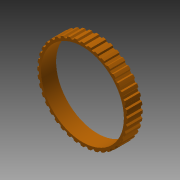
# Autodesk Inventor part: 6plactiontread
Saved by Autodesk Inventor 2013 (Build 170138000, 138)
## iProperties
Created: 2013-01-18
Part Number: 6plactiontread
Material: Rubber
Document SubType Name: Modeling
Designer: Moses
Density: 0.93 g/cm^3
Mass: 50.6346 g
Surface Area: 286.772 cm^2
Volume: 54.4458 cm^3
Author: Moses
Autodesk Inventor part; units mm, degrees
ref_plane "YZ Plane" through (0, 0, 0) normal (1, 0, 0) x (0, 1, 0)
ref_plane "XZ Plane" through (0, 0, 0) normal (0, 1, 0) x (-1, 0, 0)
ref_plane "XY Plane" through (0, 0, 0) normal (0, 0, 1) x (1, 0, 0)
sketch "Sketch1" plane through (0, 0, 0) normal (0, 0, 1) x (1, 0, 0)
  arc A0 (2.4972, 77.4343) -> (-2.4972, 77.4343) centre (0, 0) ccw
  line L0 (-3.9666, 74.7221) -> (-2.4972, 77.4343)
  line L1 (-7.7713, 74.4227) -> (-3.9666, 74.7221)
  line L2 (-9.647, 76.8716) -> (-7.7713, 74.4227)
  arc A1 (-9.647, 76.8716) -> (-14.5798, 76.0903) centre (0, 0) ccw
  line L3 (-15.6069, 73.1817) -> (-14.5798, 76.0903)
  line L4 (-19.3179, 72.2907) -> (-15.6069, 73.1817)
  line L5 (-21.5536, 74.4161) -> (-19.3179, 72.2907)
  arc A2 (-21.5536, 74.4161) -> (-26.3034, 72.8727) centre (0, 0) ccw
  line L6 (-26.8629, 69.8392) -> (-26.3034, 72.8727)
  line L7 (-30.3889, 68.3787) -> (-26.8629, 69.8392)
  line L8 (-32.9295, 70.1282) -> (-30.3889, 68.3787)
  arc A3 (-32.9295, 70.1282) -> (-37.3794, 67.8608) centre (0, 0) ccw
  line L9 (-37.4574, 64.7771) -> (-37.3794, 67.8608)
  line L10 (-40.7115, 62.783) -> (-37.4574, 64.7771)
  line L11 (-43.4945, 64.1135) -> (-40.7115, 62.783)
  arc A4 (-43.4945, 64.1135) -> (-47.535, 61.1779) centre (0, 0) ccw
  line L12 (-47.1296, 58.12) -> (-47.535, 61.1779)
  line L13 (-50.0317, 55.6414) -> (-47.1296, 58.12)
  line L14 (-52.9886, 56.5201) -> (-50.0317, 55.6414)
  arc A5 (-52.9886, 56.5201) -> (-56.5201, 52.9886) centre (0, 0) ccw
  line L15 (-55.6414, 50.0317) -> (-56.5201, 52.9886)
  line L16 (-58.12, 47.1296) -> (-55.6414, 50.0317)
  line L17 (-61.1779, 47.535) -> (-58.12, 47.1296)
  arc A6 (-61.1779, 47.535) -> (-64.1135, 43.4945) centre (0, 0) ccw
  line L18 (-62.783, 40.7115) -> (-64.1135, 43.4945)
  line L19 (-64.7771, 37.4574) -> (-62.783, 40.7115)
  line L20 (-67.8608, 37.3794) -> (-64.7771, 37.4574)
  arc A7 (-67.8608, 37.3794) -> (-70.1282, 32.9295) centre (0, 0) ccw
  line L21 (-68.3787, 30.3889) -> (-70.1282, 32.9295)
  line L22 (-69.8392, 26.8629) -> (-68.3787, 30.3889)
  line L23 (-72.8727, 26.3034) -> (-69.8392, 26.8629)
  arc A8 (-72.8727, 26.3034) -> (-74.4161, 21.5536) centre (0, 0) ccw
  line L24 (-72.2907, 19.3179) -> (-74.4161, 21.5536)
  line L25 (-73.1817, 15.6069) -> (-72.2907, 19.3179)
  line L26 (-76.0903, 14.5798) -> (-73.1817, 15.6069)
  arc A9 (-76.0903, 14.5798) -> (-76.8716, 9.647) centre (0, 0) ccw
  line L27 (-74.4227, 7.7713) -> (-76.8716, 9.647)
  line L28 (-74.7221, 3.9666) -> (-74.4227, 7.7713)
  line L29 (-77.4343, 2.4972) -> (-74.7221, 3.9666)
  arc A10 (-77.4343, 2.4972) -> (-77.4343, -2.4972) centre (0, 0) ccw
  line L30 (-74.7221, -3.9666) -> (-77.4343, -2.4972)
  line L31 (-74.4227, -7.7713) -> (-74.7221, -3.9666)
  line L32 (-76.8716, -9.647) -> (-74.4227, -7.7713)
  arc A11 (-76.8716, -9.647) -> (-76.0903, -14.5798) centre (0, 0) ccw
  line L33 (-73.1817, -15.6069) -> (-76.0903, -14.5798)
  line L34 (-72.2907, -19.3179) -> (-73.1817, -15.6069)
  line L35 (-74.4161, -21.5536) -> (-72.2907, -19.3179)
  arc A12 (-74.4161, -21.5536) -> (-72.8727, -26.3034) centre (0, 0) ccw
  line L36 (-69.8392, -26.8629) -> (-72.8727, -26.3034)
  line L37 (-68.3787, -30.3889) -> (-69.8392, -26.8629)
  line L38 (-70.1282, -32.9295) -> (-68.3787, -30.3889)
  arc A13 (-70.1282, -32.9295) -> (-67.8608, -37.3794) centre (0, 0) ccw
  line L39 (-64.7771, -37.4574) -> (-67.8608, -37.3794)
  line L40 (-62.783, -40.7115) -> (-64.7771, -37.4574)
  line L41 (-64.1135, -43.4945) -> (-62.783, -40.7115)
  arc A14 (-64.1135, -43.4945) -> (-61.1779, -47.535) centre (0, 0) ccw
  line L42 (-58.12, -47.1296) -> (-61.1779, -47.535)
  line L43 (-55.6414, -50.0317) -> (-58.12, -47.1296)
  line L44 (-56.5201, -52.9886) -> (-55.6414, -50.0317)
  arc A15 (-56.5201, -52.9886) -> (-52.9886, -56.5201) centre (0, 0) ccw
  line L45 (-50.0317, -55.6414) -> (-52.9886, -56.5201)
  line L46 (-47.1296, -58.12) -> (-50.0317, -55.6414)
  line L47 (-47.535, -61.1779) -> (-47.1296, -58.12)
  arc A16 (-47.535, -61.1779) -> (-43.4945, -64.1135) centre (0, 0) ccw
  line L48 (-40.7115, -62.783) -> (-43.4945, -64.1135)
  line L49 (-37.4574, -64.7771) -> (-40.7115, -62.783)
  line L50 (-37.3794, -67.8608) -> (-37.4574, -64.7771)
  arc A17 (-37.3794, -67.8608) -> (-32.9295, -70.1282) centre (0, 0) ccw
  line L51 (-30.3889, -68.3787) -> (-32.9295, -70.1282)
  line L52 (-26.8629, -69.8392) -> (-30.3889, -68.3787)
  line L53 (-26.3034, -72.8727) -> (-26.8629, -69.8392)
  arc A18 (-26.3034, -72.8727) -> (-21.5536, -74.4161) centre (0, 0) ccw
  line L54 (-19.3179, -72.2907) -> (-21.5536, -74.4161)
  line L55 (-15.6069, -73.1817) -> (-19.3179, -72.2907)
  line L56 (-14.5798, -76.0903) -> (-15.6069, -73.1817)
  arc A19 (-14.5798, -76.0903) -> (-9.647, -76.8716) centre (0, 0) ccw
  line L57 (-7.7713, -74.4227) -> (-9.647, -76.8716)
  line L58 (-3.9666, -74.7221) -> (-7.7713, -74.4227)
  line L59 (-2.4972, -77.4343) -> (-3.9666, -74.7221)
  arc A20 (-2.4972, -77.4343) -> (2.4972, -77.4343) centre (0, 0) ccw
  line L60 (3.9666, -74.7221) -> (2.4972, -77.4343)
  line L61 (7.7713, -74.4227) -> (3.9666, -74.7221)
  line L62 (9.647, -76.8716) -> (7.7713, -74.4227)
  arc A21 (9.647, -76.8716) -> (14.5798, -76.0903) centre (0, 0) ccw
  line L63 (15.6069, -73.1817) -> (14.5798, -76.0903)
  line L64 (19.3179, -72.2907) -> (15.6069, -73.1817)
  line L65 (21.5536, -74.4161) -> (19.3179, -72.2907)
  arc A22 (21.5536, -74.4161) -> (26.3034, -72.8727) centre (0, 0) ccw
  line L66 (26.8629, -69.8392) -> (26.3034, -72.8727)
  line L67 (30.3889, -68.3787) -> (26.8629, -69.8392)
  line L68 (32.9295, -70.1282) -> (30.3889, -68.3787)
  arc A23 (32.9295, -70.1282) -> (37.3794, -67.8608) centre (0, 0) ccw
  line L69 (37.4574, -64.7771) -> (37.3794, -67.8608)
  line L70 (40.7115, -62.783) -> (37.4574, -64.7771)
  line L71 (43.4945, -64.1135) -> (40.7115, -62.783)
  arc A24 (43.4945, -64.1135) -> (47.535, -61.1779) centre (0, 0) ccw
  line L72 (47.1296, -58.12) -> (47.535, -61.1779)
  line L73 (50.0317, -55.6414) -> (47.1296, -58.12)
  line L74 (52.9886, -56.5201) -> (50.0317, -55.6414)
  arc A25 (52.9886, -56.5201) -> (56.5201, -52.9886) centre (0, 0) ccw
  line L75 (55.6414, -50.0317) -> (56.5201, -52.9886)
  line L76 (58.12, -47.1296) -> (55.6414, -50.0317)
  line L77 (61.1779, -47.535) -> (58.12, -47.1296)
  arc A26 (61.1779, -47.535) -> (64.1135, -43.4945) centre (0, 0) ccw
  line L78 (62.783, -40.7115) -> (64.1135, -43.4945)
  line L79 (64.7771, -37.4574) -> (62.783, -40.7115)
  line L80 (67.8608, -37.3794) -> (64.7771, -37.4574)
  arc A27 (67.8608, -37.3794) -> (70.1282, -32.9295) centre (0, 0) ccw
  line L81 (68.3787, -30.3889) -> (70.1282, -32.9295)
  line L82 (69.8392, -26.8629) -> (68.3787, -30.3889)
  line L83 (72.8727, -26.3034) -> (69.8392, -26.8629)
  arc A28 (72.8727, -26.3034) -> (74.4161, -21.5536) centre (0, 0) ccw
  line L84 (72.2907, -19.3179) -> (74.4161, -21.5536)
  line L85 (73.1817, -15.6069) -> (72.2907, -19.3179)
  line L86 (76.0903, -14.5798) -> (73.1817, -15.6069)
  arc A29 (76.0903, -14.5798) -> (76.8716, -9.647) centre (0, 0) ccw
  line L87 (74.4227, -7.7713) -> (76.8716, -9.647)
  line L88 (74.7221, -3.9666) -> (74.4227, -7.7713)
  line L89 (77.4343, -2.4972) -> (74.7221, -3.9666)
  arc A30 (77.4343, -2.4972) -> (77.4343, 2.4972) centre (0, 0) ccw
  line L90 (74.7221, 3.9666) -> (77.4343, 2.4972)
  line L91 (74.4227, 7.7713) -> (74.7221, 3.9666)
  line L92 (76.8716, 9.647) -> (74.4227, 7.7713)
  arc A31 (76.8716, 9.647) -> (76.0903, 14.5798) centre (0, 0) ccw
  line L93 (73.1817, 15.6069) -> (76.0903, 14.5798)
  line L94 (72.2907, 19.3179) -> (73.1817, 15.6069)
  line L95 (74.4161, 21.5536) -> (72.2907, 19.3179)
  arc A32 (74.4161, 21.5536) -> (72.8727, 26.3034) centre (0, 0) ccw
  line L96 (69.8392, 26.8629) -> (72.8727, 26.3034)
  line L97 (68.3787, 30.3889) -> (69.8392, 26.8629)
  line L98 (70.1282, 32.9295) -> (68.3787, 30.3889)
  arc A33 (70.1282, 32.9295) -> (67.8608, 37.3794) centre (0, 0) ccw
  line L99 (64.7771, 37.4574) -> (67.8608, 37.3794)
  line L100 (62.783, 40.7115) -> (64.7771, 37.4574)
  line L101 (64.1135, 43.4945) -> (62.783, 40.7115)
  arc A34 (64.1135, 43.4945) -> (61.1779, 47.535) centre (0, 0) ccw
  line L102 (58.12, 47.1296) -> (61.1779, 47.535)
  line L103 (55.6414, 50.0317) -> (58.12, 47.1296)
  line L104 (56.5201, 52.9886) -> (55.6414, 50.0317)
  arc A35 (56.5201, 52.9886) -> (52.9886, 56.5201) centre (0, 0) ccw
  line L105 (50.0317, 55.6414) -> (52.9886, 56.5201)
  line L106 (47.1296, 58.12) -> (50.0317, 55.6414)
  line L107 (47.535, 61.1779) -> (47.1296, 58.12)
  arc A36 (47.535, 61.1779) -> (43.4945, 64.1135) centre (0, 0) ccw
  line L108 (40.7115, 62.783) -> (43.4945, 64.1135)
  line L109 (37.4574, 64.7771) -> (40.7115, 62.783)
  line L110 (37.3794, 67.8608) -> (37.4574, 64.7771)
  arc A37 (37.3794, 67.8608) -> (32.9295, 70.1282) centre (0, 0) ccw
  line L111 (30.3889, 68.3787) -> (32.9295, 70.1282)
  line L112 (26.8629, 69.8392) -> (30.3889, 68.3787)
  line L113 (26.3034, 72.8727) -> (26.8629, 69.8392)
  arc A38 (26.3034, 72.8727) -> (21.5536, 74.4161) centre (0, 0) ccw
  line L114 (19.3179, 72.2907) -> (21.5536, 74.4161)
  line L115 (15.6069, 73.1817) -> (19.3179, 72.2907)
  line L116 (14.5798, 76.0903) -> (15.6069, 73.1817)
  arc A39 (14.5798, 76.0903) -> (9.647, 76.8716) centre (0, 0) ccw
  line L117 (7.7713, 74.4227) -> (9.647, 76.8716)
  line L118 (3.9666, 74.7221) -> (7.7713, 74.4227)
  line L119 (2.4972, 77.4343) -> (3.9666, 74.7221)
  circle A40 centre (0, 0) radius 68.6967
  circle A41 centre (0, 0) radius 71.12
  dimension "d2" = 142.24
  constraints: 240 end point, 80 point on circle, 42 centre point, 1 coincident
  measures "d2" diameter of A41
extrude "Extrusion1" add sketch "Sketch1" along normal blind 25.908 contours L119 L118 L117 A39 L116 L115 L114 A38 L113 L112 L111 A37 L110 L109 L108 A36 L107 L106 L105 A35 L104 L103 L102 A34 L101 L100 L99 A33 L98 L97 L96 A32 L95 L94 L93 A31 L92 L91 L90 A30 L89 L88 L87 A29 L86 L85 L84 A28 L83 L82 L81 A27 L80 L79 L78 A26 L77 L76 L75 A25 L74 L73 L72 A24 L71 L70 L69 A23 L68 L67 L66 A22 L65 L64 L63 A21 L62 L61 L60 A20 L59 L58 L57 A19 L56 L55 L54 A18 L53 L52 L51 A17 L50 L49 L48 A16 L47 L46 L45 A15 L44 L43 L42 A14 L41 L40 L39 A13 L38 L37 L36 A12 L35 L34 L33 A11 L32 L31 L30 A10 L29 L28 L27 A9 L26 L25 L24 A8 L23 L22 L21 A7 L20 L19 L18 A6 L17 L16 L15 A5 L14 L13 L12 A4 L11 L10 L9 A3 L8 L7 L6 A2 L5 L4 L3 A1 L2 L1 L0 A0
body "Solid1"
